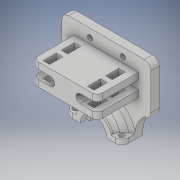
# Autodesk Inventor part: x-carriage
Saved by Autodesk Inventor 2018 (Build 220112000, 112)
## iProperties
Created: 2017-10-14
Part Number: x-carriage
Material: Generic
Document SubType Name: Modeling
Designer: Jurjen
Density: 1 g/cm^3
Appearance: Default
Author: Jurjen
Autodesk Inventor part; units mm, degrees
ref_plane "YZ Plane" through (0, 0, 0) normal (1, 0, 0) x (0, 1, 0)
ref_plane "XZ Plane" through (0, 0, 0) normal (0, 1, 0) x (-1, 0, 0)
ref_plane "XY Plane" through (0, 0, 0) normal (0, 0, 1) x (1, 0, 0)
sketch "Sketch1" plane through (0, 0, 0) normal (0, 0, 1) x (1, 0, 0)
  line L0 (-27, 15) -> (27, 15)
  line L1 (27, 15) -> (27, -15)
  line L2 (27, -15) -> (-27, -15)
  line L3 (-27, -15) -> (-27, 15)
  point P0 (0, 0)
  point P1 (0, 15)
  point P2 (-27, 0)
  dimension "d0" = 54
  dimension "d1" = 30
  constraints: 8 end point, 2 midpoint, 2 parallel, 1 horizontal, 1 horizontal alignment, 1 perpendicular, 1 vertical alignment
  measures "d0" distance between parallel lines of L1 L3
  measures "d1" distance between parallel lines of L0 L2
extrude "Extrusion1" add sketch "Sketch1" along normal mid plane 5
sketch "Sketch2" plane through (0, 0, 2.5) normal (0, 0, 1) x (1, 0, 0)
  circle A0 centre (10, 10) radius 1.6
  circle A1 centre (-10, 10) radius 1.6
  circle A2 centre (-10, -10) radius 1.6
  circle A3 centre (10, -10) radius 1.6
  line L0 (-10, 10) -> (10, 10) construction
  line L1 (-10, -10) -> (-10, 10) construction
  point P0 (0, 0)
  point P1 (0, 10)
  point P2 (-10, 0)
  dimension "d4" = 20
  dimension "d5" = 20
  dimension "d6" = 3.2
  constraints: 4 centre point, 4 end point, 3 equal radius, 3 horizontal alignment, 3 vertical alignment, 2 midpoint, 1 horizontal, 1 vertical
  measures "d4" distance of L0.end L0.start
  measures "d5" distance of L1.start L0.start
  measures "d6" diameter of A1
extrude "Extrusion2" cut sketch "Sketch2" against normal up to next
fillet "Fillet1" radius 4 4 edges at (-27, 15, 0) (-27, -15, 0) (27, -15, 0) (27, 15, 0)
sketch "Sketch3" plane through (0, 0, 2.5) normal (0, 0, 1) x (1, 0, 0)
  line L0 (-23, -15) -> (23, -15) projected
  arc A0 (8.15, -30) -> (-8.15, -30) centre (0, -30) ccw
  line L1 (17.15, -30) -> (8.15, -30)
  arc A1 (23, -15) -> (17.15, -30) centre (34.9437, -28.2988) ccw
  line L2 (0, -30) -> (0, 0) construction
  line L3 (-17.15, -30) -> (-8.15, -30)
  arc A2 (-17.15, -30) -> (-23, -15) centre (-34.9437, -28.2988) ccw
  dimension "d10" = 30
  dimension "d12" = 9
  dimension "d13" = 16.3
  constraints: 6 end point, 6 point on circle, 3 centre point, 3 symmetric about line, 1 horizontal, 1 horizontal alignment, 1 vertical, 1 vertical alignment, 1 other
  measures "d10" distance of L2.start L2.end
  measures "d12" distance of L1.start L1.end
  measures "d13" diameter of A0
extrude "Extrusion3" add sketch "Sketch3" against normal up to surface (5 mm away)
sketch "Sketch4" plane through (0, 0, 2.5) normal (0, 0, 1) x (1, 0, 0)
  arc A0 (8.15, -30) -> (-8.15, -30) centre (0, -30) ccw projected
  arc A1 (6.25, -30) -> (-6.25, -30) centre (0, -30) ccw
  line L0 (-6.25, -30) -> (-17.15, -30)
  arc A2 (-17.15, -30) -> (-23, -15) centre (-34.9437, -28.2988) ccw projected
  line L1 (17.15, -30) -> (8.15, -30) projected
  line L2 (17.15, -30) -> (6.25, -30)
  arc A3 (8.15, -30) -> (-8.15, -30) centre (0, -30) ccw
  point P0 (0, 0)
  dimension "d16" = 12.5
  constraints: 6 point on circle, 4 end point, 2 centre point, 2 coincident, 2 point on line, 1 collinear, 1 horizontal alignment
  measures "d16" diameter of A1
extrude "Extrusion4" add sketch "Sketch4" along normal blind 3.8 and the other way blind 1.8
sketch "Sketch5" plane through (0, 0, 2.5) normal (0, 0, 1) x (1, 0, 0)
  arc A0 (27, 11) -> (23, 15) centre (23, 11) ccw projected
  line L0 (23, 15) -> (-23, 15) projected
  arc A1 (-23, 15) -> (-27, 11) centre (-23, 11) ccw projected
  line L1 (-27, 11) -> (-27, -11) projected
  arc A2 (-27, -11) -> (-23, -15) centre (-23, -11) ccw projected
  arc A3 (-17.15, -30) -> (-23, -15) centre (-34.9437, -28.2988) ccw projected
  line L2 (-8.15, -30) -> (-17.15, -30) projected
  arc A4 (8.15, -30) -> (-8.15, -30) centre (0, -30) ccw projected
  line L3 (17.15, -30) -> (8.15, -30) projected
  arc A5 (23, -15) -> (17.15, -30) centre (34.9437, -28.2988) ccw projected
  arc A6 (23, -15) -> (27, -11) centre (23, -11) ccw projected
  line L4 (27, -11) -> (27, 11) projected
  circle A7 centre (-10, -10) radius 1.6 projected
  circle A8 centre (10, 10) radius 1.6 projected
  circle A9 centre (-10, 10) radius 1.6 projected
  circle A10 centre (10, -10) radius 1.6 projected
  arc A11 (23, -15) -> (17.15, -30) centre (34.9437, -28.2988) ccw projected
  line L5 (17.1161, -27) -> (7.5778, -27)
  line L6 (-7.5778, -27) -> (-17.1161, -27)
  point P0 (0, 0)
  dimension "d21" = 3
  constraints: 4 end point, 4 point on circle, 2 point on line, 1 horizontal
  measures "d21" distance between parallel lines of L3 L5
extrude "Extrusion5" add sketch "Sketch5" along normal up to surface (3.8 mm away) contours A5 L3 A4 L5 | A4 L2 A3 L6
sketch "Sketch6" plane through (0, 0, 6.3) normal (0, 0, 1) x (1, 0, 0)
  arc A0 (8.15, -30) -> (-8.15, -30) centre (0, -30) ccw projected
  arc A1 (8.15, -30) -> (-8.15, -30) centre (0, -30) ccw
  arc A2 (11.15, -30) -> (-11.15, -30) centre (0, -30) ccw
  arc A3 (6.25, -30) -> (-6.25, -30) centre (0, -30) ccw projected
  line L0 (-6.25, -30) -> (-17.15, -30) projected
  line L1 (-6.25, -30) -> (-17.15, -30)
  line L2 (6.25, -30) -> (12.2947, -30)
  point P0 (0, 0)
  dimension "d24" = 3
  constraints: 6 point on circle, 4 end point, 4 point on line, 2 centre point, 2 coincident, 2 horizontal
  measures "d24" radial gap between concentric circles of A2 A1
extrude "Extrusion6" add sketch "Sketch6" along normal blind 4 contours A0 L0 A2 L2
sketch "Sketch9" plane through (0, 0, 6.3) normal (0, 0, 1) x (1, 0, 0)
  arc A0 (-10.7388, -27) -> (-11.15, -30) centre (0, -30) ccw projected
  line L0 (-17.1161, -27) -> (-10.7388, -27) projected
  arc A1 (-17.15, -30) -> (-17.1161, -27) centre (-34.9437, -28.2988) ccw projected
  line L1 (-11.15, -30) -> (-17.15, -30) projected
  arc A2 (11.15, -30) -> (10.7388, -27) centre (0, -30) ccw projected
  line L2 (11.15, -30) -> (17.15, -30) projected
  arc A3 (17.1161, -27) -> (17.15, -30) centre (34.9437, -28.2988) ccw projected
  line L3 (10.7388, -27) -> (17.1161, -27) projected
  point P0 (0, 0)
extrude "Extrusion7" add sketch "Sketch9" along normal up to surface (4 mm away)
sketch "Sketch10" plane through (0, 0, 6.3) normal (0, 0, -1) x (-1, 0, 0)
  line L0 (10.7388, -27) -> (7.5778, -27) projected
  arc A0 (10.7388, -27) -> (-10.7388, -27) centre (0, -30) ccw projected
  line L1 (-7.5778, -27) -> (-10.7388, -27) projected
  arc A1 (7.5778, -27) -> (-7.5778, -27) centre (0, -30) ccw projected
  point P0 (0, 0)
extrude "Extrusion8" add sketch "Sketch10" along normal up to surface (3.8 mm away)
chamfer "Chamfer1" distance 5 angle 45 1 edges at (0, -18.85, 2.5)
fillet "Fillet2" radius 4 2 edges at (17.07, -28.5007, 10.3) (-17.07, -28.5007, 10.3)
fillet "Fillet3" radius 4 2 edges at (0, -18.85, 7.5) (0, -13.85, 2.5)
sketch "Sketch13" plane through (-17.15, -30, -2.5) normal (0, -1, 0) x (1, 0, 0)
  circle A0 centre (3, 9.8) radius 1.6
  circle A1 centre (31.3, 9.8) radius 1.6
  line L0 (0, 0) -> (0, 8.8) projected
  line L1 (9, 12.8) -> (4.0149, 12.8) projected
  line L2 (34.3, 8.8) -> (34.3, 0) projected
  point P0 (17.15, 2.5)
  dimension "d45" = 3.2
  dimension "d46" = 3
  dimension "d47" = 3
  dimension "d48" = 3
  constraints: 2 centre point, 1 equal radius, 1 horizontal alignment
  measures "d45" diameter of A0
  measures "d46" distance from line of A0.centre L0
  measures "d47" distance from line of L1 A0.centre
  measures "d48" distance from line of A1.centre L2
extrude "Extrusion10" cut sketch "Sketch13" against normal up to next
sketch "Sketch14" plane through (0, 0, 2.5) normal (0, 0, 1) x (1, 0, 0)
  line L0 (19.5, 6.65) -> (-19.5, 6.65)
  line L1 (-19.5, 6.65) -> (-19.5, 2.65)
  line L2 (-19.5, 2.65) -> (-6.5, 2.65)
  line L3 (-6.5, 2.65) -> (-6.5, -2.65)
  line L4 (-6.5, -2.65) -> (-19.5, -2.65)
  line L5 (-19.5, -2.65) -> (-19.5, -6.65)
  line L6 (-19.5, -6.65) -> (19.5, -6.65)
  line L7 (19.5, -6.65) -> (19.5, -2.65)
  line L8 (19.5, -2.65) -> (6.5, -2.65)
  line L9 (6.5, -2.65) -> (6.5, 2.65)
  line L10 (6.5, 2.65) -> (19.5, 2.65)
  line L11 (19.5, 6.65) -> (19.5, 2.65)
  point P0 (0, 0)
  point P1 (0, 6.65)
  point P2 (0, -6.65)
  point P3 (6.5, 0)
  point P4 (-6.5, 0)
  dimension "d51" = 4
  dimension "d52" = 4
  dimension "d53" = 5.3
  dimension "d54" = 13
  dimension "d55" = 39
  dimension "d56" = 13
  constraints: 24 end point, 9 perpendicular, 5 point on line, 4 midpoint, 2 horizontal alignment, 2 vertical alignment, 1 horizontal
  measures "d51" distance between parallel lines of L10 L0
  measures "d52" distance between parallel lines of L6 L8
  measures "d53" distance between parallel lines of L8 L10
  measures "d54" distance between parallel lines of L9 L11
  measures "d55" distance between parallel lines of L1 L11
  measures "d56" distance between parallel lines of L1 L3
extrude "Extrusion11" add sketch "Sketch14" along normal blind 25
sketch "Sketch15" plane through (-19.5, -6.65, 2.5) normal (0, -1, 0) x (1, 0, 0)
  line L0 (4, 23) -> (8, 23)
  line L1 (8, 23) -> (8, 15)
  line L2 (8, 15) -> (4, 15)
  line L3 (4, 15) -> (4, 23)
  line L4 (4, 12) -> (8, 12)
  line L5 (8, 12) -> (8, 4)
  line L6 (8, 4) -> (4, 4)
  line L7 (4, 4) -> (4, 12)
  line L8 (0, 25) -> (39, 25) projected
  line L9 (0, 0) -> (0, 25) projected
  point P0 (19.5, -2.5)
  dimension "d59" = 4
  dimension "d60" = 8
  dimension "d61" = 8
  dimension "d62" = 2
  dimension "d63" = 3
  dimension "d64" = 4
  constraints: 16 end point, 4 parallel, 2 horizontal, 2 perpendicular, 1 point on line, 1 vertical alignment
  measures "d59" distance between parallel lines of L1 L3
  measures "d60" distance between parallel lines of L0 L2
  measures "d61" distance between parallel lines of L6 L4
  measures "d62" distance between parallel lines of L8 L0
  measures "d63" distance between parallel lines of L4 L2
  measures "d64" distance between parallel lines of L9 L3
extrude "Extrusion12" cut sketch "Sketch15" against normal blind 20
fillet "Fillet4" radius 2.5 4 edges at (-6.5, -2.65, 15) (-6.5, 2.65, 15) (6.5, 2.65, 15) (6.5, -2.65, 15)
mirror "Mirror1" about plane through (0, 0, 0) normal (1, 0, 0) of "Extrusion12"
fillet "Fillet5" radius 3 4 edges at (-19.5, -4.65, 27.5) (-19.5, 4.65, 27.5) (19.5, 4.65, 27.5) (19.5, -4.65, 27.5)
body "Solid1"
